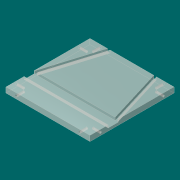
# Autodesk Inventor part: topBottom
Saved by Autodesk Inventor 2016 (Build 200138000, 138)
## iProperties
Created: 2015-10-13
Part Number: topBottom
Material: PC/ABS Plastic
Document SubType Name: Modeling
Designer: Sawaiz
Density: 0.357273 g/cm^3
Appearance: Clear
Author: Sawaiz
Autodesk Inventor part; units mm, degrees
ref_plane "YZ Plane" through (0, 0, 0) normal (1, 0, 0) x (0, 1, 0)
ref_plane "XZ Plane" through (0, 0, 0) normal (0, 1, 0) x (-1, 0, 0)
ref_plane "XY Plane" through (0, 0, 0) normal (0, 0, 1) x (1, 0, 0)
sketch "Sketch1" plane through (0, 0, 0) normal (0, 0, 1) x (1, 0, 0)
  line L0 (-50, -50) -> (50, -50)
  line L1 (50, -50) -> (50, 50)
  line L2 (50, 50) -> (-50, 50)
  line L3 (-50, 50) -> (-50, -50)
  line L4 (-50, -50) -> (50, 50) construction
  line L5 (50, -50) -> (-50, 50) construction
  point P0 (0, 0)
  dimension "d0" = 100
  dimension "d1" = 100
  constraints: 12 end point, 2 midpoint, 2 parallel, 1 horizontal, 1 perpendicular
  measures "d0" distance of L2.end L1.end
  measures "d1" distance of L1.end L0.end
extrude "Extrusion1" add sketch "Sketch1" along normal blind 6.35
sketch "Sketch3" plane through (0, 0, 6.35) normal (0, 0, 1) x (1, 0, 0)
  line L0 (-50, -50) -> (50, -50) projected
  line L1 (50, -50) -> (50, 50) projected
  line L2 (50, 50) -> (-50, 50) projected
  line L3 (-50, 50) -> (-50, -50) projected
  line L4 (-50, -50) -> (50, -50) projected
  line L5 (28.376, -53.1371) -> (-50, -29.1751)
  line L6 (28.376, -50) -> (-50, -26.0381)
  line L7 (-50, 26.0381) -> (28.376, 50)
  line L8 (50, -50) -> (50, 50) projected
  line L9 (28.376, 53.1371) -> (-50, 29.1751)
  line L10 (50, 50) -> (-50, 50) projected
  line L11 (-50, 50) -> (-50, -50) projected
  line L12 (-50, -26.0381) -> (-50, 26.0381)
  line L13 (28.376, 53.1371) -> (28.376, -53.1371)
  point P0 (0, 0)
  point P1 (-50, 0)
  dimension "d10" = 3
  dimension "d11" = 3
  dimension "d16" = 21.624
  dimension "d17" = 17
  dimension "d18" = 81.9571
  constraints: 12 end point, 9 point on line, 2 midpoint, 2 parallel, 1 collinear, 1 vertical
  measures "d10" distance between parallel lines of L7 L9
  measures "d11" distance between parallel lines of L5 L6
  measures "d16" distance between parallel lines of L1 L13
  measures "d17" angle of L0 L6
  measures "d18" distance of L7.start L7.end
extrude "Extrusion2" cut sketch "Sketch3" against normal blind 3.175 contours L13 L5 L0 | L0 L5 L3 L6 | L7 L3 L9 L2 | L2 L9 L13
sketch "Sketch4" plane through (0, 0, 6.35) normal (0, 0, 1) x (1, 0, 0)
  line L0 (50, -50) -> (50, 50) projected
  line L1 (28.376, -50) -> (50, -50) projected
  line L2 (50, 50) -> (28.376, 50) projected
  line L3 (-50, -26.0381) -> (28.376, -50) projected
  line L4 (28.376, -50) -> (16.376, -50)
  line L5 (16.376, -50) -> (16.376, 50)
  line L6 (16.376, 50) -> (28.376, 50)
  line L7 (28.376, 50) -> (28.376, -50)
  point P0 (0, 0)
  dimension "d19" = 12
  constraints: 8 end point, 2 parallel, 1 horizontal, 1 perpendicular
  measures "d19" distance between parallel lines of L5 L7
extrude "Extrusion3" cut sketch "Sketch4" against normal blind 3.175 contours L4 L5 L3 | L3 L5 L6 L7
sketch "Sketch5" plane through (-50, 50, 0) normal (0, 1, 0) x (1, 0, 0)
  line L0 (66.376, -6.35) -> (66.376, -3.175) projected
  line L1 (66.376, -3.175) -> (78.376, -3.175) projected
  line L2 (78.376, -3.175) -> (78.376, -6.35) projected
  line L3 (100, -6.35) -> (78.376, -6.35) projected
  line L4 (100, 0) -> (100, -6.35) projected
  line L5 (100, 0) -> (0, 0) projected
  line L6 (0, 0) -> (0, -6.35) projected
  line L7 (66.376, -6.35) -> (0, -6.35) projected
  line L8 (100, -3.175) -> (0, -3.175)
  line L9 (0, -3.175) -> (66.376, -3.175) projected
  point P0 (50, 0)
  point P1 (62.5, -3.175)
  point P2 (37.5, -3.175)
  point P3 (12.5, -3.175)
  point P4 (87.5, -3.175)
  dimension "d22" = 3.175
  dimension "d23" = 12.5
  dimension "d24" = 12.5
  dimension "d25" = 25
  dimension "d26" = 25
  constraints: 4 point on line, 2 end point, 2 midpoint, 1 horizontal
  measures "d22" distance between parallel lines of L5 L8
  measures "d23" horizontal distance of point (50, 0) point (62.5, -3.175)
  measures "d24" horizontal distance of point (50, 0) point (37.5, -3.175)
  measures "d25" distance of point (37.5, -3.175) point (12.5, -3.175)
  measures "d26" distance of point (87.5, -3.175) point (62.5, -3.175)
hole "Hole1" at (-37.5, 50, 3.175) at (37.5, 50, 3.175) direction (0, -1, 0) diameter 2.459 depth 8.8 tip angle 118 thread size "M3x0.5" class "6H" standard "ANSI Metric M Profile"
mirror "Mirror1" about plane through (0, 0, 0) normal (0, 1, 0) of "Hole1"
sketch "Sketch6" plane through (50, -50, 0) normal (1, 0, 0) x (0, 0, -1)
  line L0 (0, 0) -> (0, 100) projected
  line L1 (0, 100) -> (-6.35, 100) projected
  line L2 (-6.35, 0) -> (-6.35, 100) projected
  line L3 (0, 0) -> (-6.35, 0) projected
  line L4 (-3.175, 0) -> (-3.175, 100)
  line L5 (-3.175, 3.6688) -> (-3.175, 96.3312) projected
  point P0 (0, 50)
  point P1 (-3.175, 12.5)
  point P2 (-3.175, 37.5)
  point P3 (-3.175, 62.5)
  point P4 (-3.175, 87.5)
  dimension "d34" = 3.175
  dimension "d35" = 12.5
  dimension "d36" = 12.5
  dimension "d37" = 25
  dimension "d38" = 25
  constraints: 4 point on line, 2 end point, 2 midpoint, 1 vertical
  measures "d34" distance between parallel lines of L2 L4
  measures "d35" vertical distance of point (-3.175, 62.5) point (0, 50)
  measures "d36" vertical distance of point (-3.175, 37.5) point (0, 50)
  measures "d37" distance of point (-3.175, 37.5) point (-3.175, 12.5)
  measures "d38" distance of point (-3.175, 62.5) point (-3.175, 87.5)
hole "Hole2" at (50, -37.5, 3.175) at (50, 37.5, 3.175) direction (-1, 0, 0) diameter 2.459 depth 8.8 tip angle 118 thread size "M3x0.5" class "6H" standard "ANSI Metric M Profile"
mirror "Mirror2" about plane through (0, 0, 0) normal (1, 0, 0) of "Hole2"
equation "\"d0\" = depth"
equation "\"d1\" = width"
equation "\"d2\" = acrylicThickness"
equation "\"d10\" = mirrorThickness"
equation "\"d11\" = mirrorThickness"
equation "\"d16\" = centerThickness + aerogelThickness + fresnelThickness"
equation "\"d17\" = mirrorAngle"
equation "\"d7\" = 0.5 * acrylicThickness"
equation "\"d19\" = 4 * mirrorThickness"
equation "\"d20\" = 0.5 * acrylicThickness"
equation "\"d22\" = 0.5 * acrylicThickness"
equation "\"d23\" = 0.125 * depth"
equation "\"d24\" = 0.125 * depth"
equation "\"d25\" = 0.25 * depth"
equation "\"d26\" = 0.25 * depth"
equation "\"d34\" = 0.5 * acrylicThickness"
equation "\"d35\" = 0.125 * width"
equation "\"d36\" = 0.125 * width"
equation "\"d37\" = 0.25 * width"
equation "\"d38\" = 0.25 * width"
equation "\"acrylicThickness\" = 6.35"
equation "\"width\" = 100"
equation "\"depth\" = 100"
equation "\"mirrorAngle\" = 17deg"
equation "\"mirrorThickness\" = 3"
equation "\"aerogelThickness\" = 20"
equation "\"detectorWidth\" = 52"
equation "\"detectorHeight\" = 52"
equation "\"fresnelThickness\" = 0.1"
equation "\"focalLength\" = 76.2"
equation "\"ior\" = 1.49"
equation "\"centerThickness\" = 1.524"
equation "\"fresnelAngle\" = 90deg"
equation "\"fresnelEffectiveDiameter\" = 76.2"
body "Solid1"
